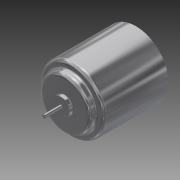
# Autodesk Inventor part: Motor
Saved by Autodesk Inventor 2013 (Build 170138000, 138)
## iProperties
Created: 2013-06-27
Part Number: Motor
Material: Generic
Document SubType Name: Modeling
Designer: Kyle
Density: 1 g/cm^3
Author: Kyle
Autodesk Inventor part; units mm, degrees
ref_plane "YZ Plane" through (0, 0, 0) normal (1, 0, 0) x (0, 1, 0)
ref_plane "XZ Plane" through (0, 0, 0) normal (0, 1, 0) x (-1, 0, 0)
ref_plane "XY Plane" through (0, 0, 0) normal (0, 0, 1) x (1, 0, 0)
sketch "Sketch1" plane through (0, 0, 0) normal (0, 0, 1) x (1, 0, 0)
  circle A0 centre (0, 0) radius 12.065
  dimension "d0" = 24.13
  constraints: 1 centre point, 1 coincident
  measures "d0" diameter of A0
extrude "Extrusion1" add sketch "Sketch1" along normal blind 24.13
sketch "Sketch2" plane through (0, 0, 24.13) normal (0, 0, 1) x (1, 0, 0)
  circle A0 centre (0, 0) radius 12.065 projected
  circle A1 centre (0, 0) radius 9.525
  dimension "d4" = 19.05
  constraints: 1 centre point, 1 coincident
  measures "d4" diameter of A1
extrude "Extrusion2" add sketch "Sketch2" along normal blind 2.54 contours A1
sketch "Sketch3" plane through (0, 0, 26.67) normal (0, 0, 1) x (1, 0, 0)
  circle A0 centre (0, 0) radius 9.525 projected
  circle A1 centre (0, 0) radius 3.175
  dimension "d8" = 6.35
  constraints: 1 centre point, 1 coincident
  measures "d8" diameter of A1
extrude "Extrusion3" add sketch "Sketch3" along normal blind 1.27 contours A1
sketch "Sketch4" plane through (0, 0, 27.94) normal (0, 0, 1) x (1, 0, 0)
  circle A0 centre (0, 0) radius 3.175 projected
  circle A1 centre (0, 0) radius 0.635
  dimension "d12" = 1.27
  constraints: 1 centre point, 1 coincident
  measures "d12" diameter of A1
extrude "Extrusion4" add sketch "Sketch4" along normal blind 6.35 contours A1
fillet "Fillet1" radius 1.27 2 edges at (-12.065, 0, 24.13) (-9.525, 0, 26.67)
fillet "Fillet2" radius 0.635 1 edges at (-9.525, 0, 24.13)
fillet "Fillet3" radius 0.254 1 edges at (-3.175, 0, 26.67)
body "Solid1"
